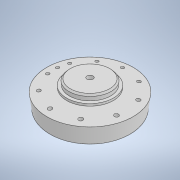
# Autodesk Inventor part: bottom
Saved by Autodesk Inventor 2022 (Build 260153000, 153)
## iProperties
Created: 2022-06-04
Part Number: bottom
Material: Generic
Document SubType Name: Modeling
Designer: Jacob
Density: 1 g/cm^3
Appearance: Default
Author: Jacob
Autodesk Inventor part; units mm, degrees
ref_plane "YZ Plane" through (0, 0, 0) normal (1, 0, 0) x (0, 1, 0)
ref_plane "XZ Plane" through (0, 0, 0) normal (0, 1, 0) x (-1, 0, 0)
ref_plane "XY Plane" through (0, 0, 0) normal (0, 0, 1) x (1, 0, 0)
sketch "Sketch1" plane through (0, 0, 0) normal (0, 1, 0) x (-1, 0, 0)
  circle A0 centre (0, 0) radius 30
  dimension "d0" = 60
  constraints: 1 centre point, 1 coincident
  measures "d0" diameter of A0
extrude "Extrusion1" add sketch "Sketch1" along normal blind 10
sketch "Sketch2" plane through (0, 10, 0) normal (0, 1, 0) x (1, 0, 0)
  circle A0 centre (0, 0) radius 14.245
  dimension "d3" = 28.49
  constraints: 1 centre point, 1 coincident
  measures "d3" diameter of A0
extrude "Extrusion2" add sketch "Sketch2" along normal blind 5
sketch "Sketch3" plane through (0, 10, 0) normal (0, 1, 0) x (1, 0, 0)
  circle A0 centre (-25.3377, 0) radius 1.27
  point P0 (0, 0)
  dimension "d6" = 2.54
  dimension "d7" = 25.3377
  constraints: 1 centre point
  measures "d6" diameter of A0
  measures "d7" distance of point (0, 0) A0.centre
extrude "Extrusion3" cut sketch "Sketch3" against normal up to surface (10 mm away)
sketch "Sketch4" plane through (0, 15, 0) normal (0, 1, 0) x (1, 0, 0)
  circle A0 centre (0, 0) radius 2.1
  dimension "d10" = 4.2
  constraints: 1 centre point, 1 coincident
  measures "d10" diameter of A0
extrude "Extrusion4" cut sketch "Sketch4" against normal up to surface (15 mm away)
chamfer "Chamfer1" distance 1 angle 45 1 edges at (-14.245, 15, 0)
sketch "Sketch6" plane through (0, 10, 0) normal (0, 1, 0) x (1, 0, 0)
  circle A0 centre (-25.3377, 0) radius 1.27 projected
  circle A1 centre (-25.3377, 0) radius 1.27 projected
  line L0 (-25.3377, 0) -> (0, 0) construction
  line L1 (0, 0) -> (-24.0976, 7.8298) construction
  circle A2 centre (0, 0) radius 25.3377 construction
  circle A3 centre (-24.0976, 7.8298) radius 1.27
  circle A4 centre (-24.0976, -7.8298) radius 1.27
  circle A5 centre (-14.8931, -20.4986) radius 1.27
  circle A6 centre (0, -25.3377) radius 1.27
  circle A7 centre (14.8931, -20.4986) radius 1.27
  circle A8 centre (24.0976, -7.8298) radius 1.27
  circle A9 centre (24.0976, 7.8298) radius 1.27
  circle A10 centre (14.8931, 20.4986) radius 1.27
  circle A11 centre (0, 25.3377) radius 1.27
  circle A12 centre (-14.8931, 20.4986) radius 1.27
  point P0 (-24.9704, -1.2157)
  point P1 (-24.9704, 1.2157)
  dimension "d22" = 18
  dimension "d23" = 2.54
  dimension "d24" = 2.54
  dimension "d27" = 360
  constraints: 11 centre point, 4 end point, 2 coincident, 2 point on circle, 1 horizontal, 21 other
  measures "d22" angle of L0 L1
  measures "d23" diameter of A0
  measures "d24" diameter of A3
extrude "Extrusion6" cut sketch "Sketch6" against normal up to surface (10 mm away) contours A3 | A4 | A5 | A6 | A7 | A8 | A9 | A10 | A11 | A12
sketch "Sketch7" plane through (0, 10, 0) normal (0, 1, 0) x (1, 0, 0)
  circle A0 centre (0, 0) radius 14.245 projected
  circle A1 centre (0, 0) radius 16.245
  dimension "d31" = 2
  constraints: 1 centre point
  measures "d31" radial gap between concentric circles of A0 A1
extrude "Extrusion7" add sketch "Sketch7" along normal blind 1.5
sketch "Sketch8" plane through (0, 10, 0) normal (0, 1, 0) x (1, 0, 0)
  circle A0 centre (0, 0) radius 16.245 projected
  circle A1 centre (0, -25.3377) radius 1.27 projected
  circle A2 centre (-24.0976, -7.8298) radius 1.27 projected
  circle A3 centre (-14.8931, 20.4986) radius 1.27 projected
  circle A4 centre (24.0976, -7.8298) radius 1.27 projected
  circle A5 centre (24.0976, 7.8298) radius 1.27 projected
  circle A6 centre (-24.0976, 7.8298) radius 1.27 projected
  circle A7 centre (-14.8931, -20.4986) radius 1.27 projected
  circle A8 centre (0, 25.3377) radius 1.27 projected
  circle A9 centre (14.8931, -20.4986) radius 1.27 projected
  circle A10 centre (14.8931, 20.4986) radius 1.27 projected
  circle A11 centre (-25.3377, 0) radius 1.27 projected
  circle A12 centre (0, 0) radius 30 projected
  circle A13 centre (0, 0) radius 16.245 projected
  circle A14 centre (0, 0) radius 14.245 projected
equation "\"d24\" = d23"
body "Solid1"
